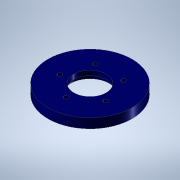
# Autodesk Inventor part: OutputShaft
Saved by Autodesk Inventor 2021 (Build 250183000, 183)
## iProperties
Created: 2022-08-31
Part Number: OutputShaft
Material: Ogólny
Document SubType Name: Modeling
Designer: MicnedSQ
Density: 1 g/cm^3
Appearance: Domyślna
Author: MicnedSQ
## iProperties of the stored document _Drukowanie 3D.ipt
Created: 2022-09-01
Part Number: _Drukowanie 3D
Material: Ogólny
Document SubType Name: Modeling
Designer: MicnedSQ
Density: 1 g/cm^3
Appearance: Domyślna
Author: MicnedSQ
Autodesk Inventor part; units mm, degrees
ref_plane "YZ Plane" through (0, 0, 0) normal (1, 0, 0) x (0, 1, 0)
ref_plane "XZ Plane" through (0, 0, 0) normal (0, 1, 0) x (-1, 0, 0)
ref_plane "XY Plane" through (0, 0, 0) normal (0, 0, 1) x (1, 0, 0)
sketch "Szkic1" plane through (0, 0, 0) normal (0, 1, 0) x (-1, 0, 0)
  circle A0 centre (0, 0) radius 35
  dimension "d0" = 70
  constraints: 1 centre point, 1 coincident
  measures "d0" diameter of A0
extrude "Wyciągnięcie proste1" add sketch "Szkic1" along normal blind 8
sketch "Szkic2" plane through (0, 0, 0) normal (0, -1, 0) x (1, 0, 0)
  circle A0 centre (0, 0) radius 28
  circle A1 centre (28, 0) radius 5
  dimension "d3" = 56
  dimension "d4" = 10
  constraints: 1 centre point, 1 coincident, 1 horizontal alignment, 2 other
  measures "d4" diameter of A1
sketch "Szkic3" plane through (0, 0, 0) normal (0, -1, 0) x (1, 0, 0)
  circle A0 centre (0, 0) radius 16.1
  dimension "d9" = 32.2
  constraints: 1 centre point, 1 coincident
  measures "d9" diameter of A0
extrude "Wyciągnięcie proste2" cut sketch "Szkic3" against normal blind 4
extrude "Wyciągnięcie proste3" add sketch "Szkic2" along normal blind 1.5 contours A0 A1 | A0 A1 picked at (26.3673, 0.9633) picked at (29.4661, 1.3172)
pattern_circular "Szyk kołowy1" count 10 over 360 about axis through (0, 0, 0) along (0, 1, 0) of "Wyciągnięcie proste3"
sketch "Szkic4" plane through (0, 4, 0) normal (0, -1, 0) x (1, 0, 0)
  circle A0 centre (0, 0) radius 13.5
  dimension "d17" = 27
  constraints: 1 centre point, 1 coincident
  measures "d17" diameter of A0
extrude "Wyciągnięcie proste4" cut sketch "Szkic4" against normal blind 4
sketch "Szkic5" plane through (28, -1.5, 0) normal (0, -1, 0) x (1, 0, 0)
  circle A0 centre (0, 0) radius 5 projected
  circle A1 centre (0, 0) radius 1.4
  point P0 (-28, 0)
  dimension "d20" = 2.8
  constraints: 1 centre point, 1 coincident
  measures "d20" diameter of A1
extrude "Wyciągnięcie proste5" cut sketch "Szkic5" against normal blind 6 contours A1
pattern_circular "Szyk kołowy2" count 10 over 360 about axis through (0, 0, 0) along (0, 1, 0) of "Wyciągnięcie proste5"
sketch "Szkic6" plane through (0, 8, 0) normal (0, 1, 0) x (1, 0, 0)
  circle A0 centre (0, 0) radius 20
  circle A1 centre (0, -20) radius 1.9
  dimension "d26" = 40
  dimension "d27" = 3.8
  constraints: 1 centre point, 1 coincident, 1 vertical alignment, 2 other
  measures "d27" diameter of A1
extrude "Wyciągnięcie proste6" cut sketch "Szkic6" against normal blind 6 contours A1 A0 | A0 A1 picked at (0.074, -19.3643) picked at (0.0625, -20.6235)
pattern_circular "Szyk kołowy3" count 5 over 360 about axis through (0, 4, 0) along (0, 1, 0) of "Wyciągnięcie proste6"
